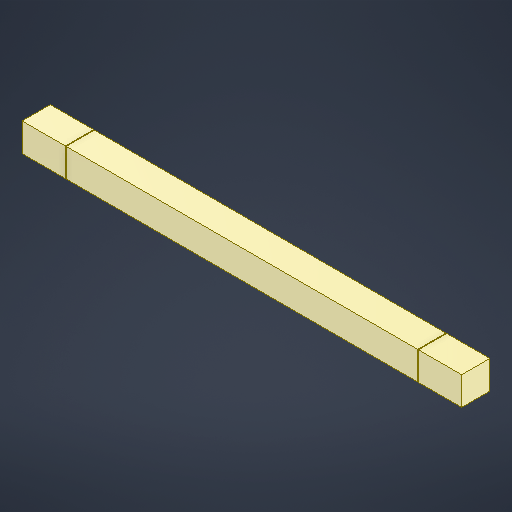
# Autodesk Inventor part: Torsion
Saved by Autodesk Inventor 2025 (Build 290162000, 162)
## iProperties
Created: 2024-12-26
Part Number: Torsion
Material: Нейлон 6/6
Document SubType Name: Modeling
Designer: khrip
Density: 1.13 g/cm^3
Appearance: Нейлон 6
Author: khrip
Autodesk Inventor part; units mm, degrees
ref_plane "YZ Plane" through (0, 0, 0) normal (1, 0, 0) x (0, 1, 0)
ref_plane "XZ Plane" through (0, 0, 0) normal (0, 1, 0) x (-1, 0, 0)
ref_plane "XY Plane" through (0, 0, 0) normal (0, 0, 1) x (1, 0, 0)
sketch "Эскиз1" plane through (0, 0, 0) normal (1, 0, 0) x (0, 1, 0)
  line L0 (2.25, -2.25) -> (-2.25, -2.25)
  line L1 (-2.25, -2.25) -> (-2.25, 2.25)
  line L2 (-2.25, 2.25) -> (2.25, 2.25)
  line L3 (2.25, 2.25) -> (2.25, -2.25)
  line L4 (2.25, -2.25) -> (-2.25, 2.25) construction
  line L5 (-2.25, -2.25) -> (2.25, 2.25) construction
  point P0 (0, 0)
  dimension "d0" = 4.5
  dimension "d1" = 4.5
  constraints: 12 end point, 2 midpoint, 2 parallel, 1 horizontal, 1 perpendicular
  measures "d0" distance of L1.end L2.end
  measures "d1" distance of L0.end L1.end
extrude "Выдавливание1" add sketch "Эскиз1" along normal blind 70
sketch "Эскиз2" plane through (0, -2.25, 2.25) normal (0, 0, 1) x (1, 0, 0)
  line L0 (0, 4.5) -> (0, 0) projected
  line L1 (0, 0) -> (70, 0) projected
  line L2 (70, 4.5) -> (70, 0) projected
  line L3 (0, 4.5) -> (70, 4.5) projected
  line L4 (6.9, 4.5) -> (7, 4.5)
  line L5 (7, 4.5) -> (7, 0)
  line L6 (7, 0) -> (6.9, 0)
  line L7 (6.9, 0) -> (6.9, 4.5)
  line L8 (63, 4.5) -> (63.1, 4.5)
  line L9 (63.1, 4.5) -> (63.1, 0)
  line L10 (63.1, 0) -> (63, 0)
  line L11 (63, 0) -> (63, 4.5)
  point P0 (0, 2.25)
  point P1 (63, 0)
  point P2 (6.9, 0)
  dimension "d4" = 0.1
  dimension "d5" = 0.1
  dimension "d6" = 6.9
  dimension "d7" = 6.9
  constraints: 16 end point, 4 parallel, 4 point on line, 2 horizontal, 2 perpendicular
  measures "d4" distance of L5.end L6.end
  measures "d5" distance of L9.end L10.end
  measures "d6" distance between parallel lines of L2 L9
  measures "d7" distance between parallel lines of L0 L7
extrude "Выдавливание2" cut sketch "Эскиз2" against normal blind 0.1 contours L3 L5 L1 L7 | L3 L9 L1 L11
pattern_circular "Круговой массив1" count 4 over 360 about axis through (-10, 0, 0) along (1, 0, 0) of "Выдавливание2"
sketch "Эскиз3" plane through (70, 0, 0) normal (1, 0, 0) x (0, 0, -1)
  line L0 (-2.25, 2.25) -> (-2.25, -2.25) projected
  line L1 (-2.25, -2.25) -> (2.25, -2.25) projected
  line L2 (2.25, -2.25) -> (2.25, 2.25) projected
  line L3 (2.25, 2.25) -> (-2.25, 2.25) projected
  point P0 (0, 0)
  constraints: 1 coincident, 3 other
